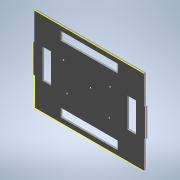
# Autodesk Inventor part: Level3
Saved by Autodesk Inventor 2020 (Build 240168000, 168)
## iProperties
Part Number: Level3
Material: Generic
Document SubType Name: Modeling
Designer: SBBA
Appearance: Default
Mass: 74.2606 g
Surface Area: 539.274 cm^2
Volume: 74.2606 cm^3
Density: 1 g/cm^3
Author: SBBA
Autodesk Inventor part; units mm, degrees
ref_plane "YZ Plane" through (0, 0, 0) normal (1, 0, 0) x (0, 1, 0)
ref_plane "XZ Plane" through (0, 0, 0) normal (0, 1, 0) x (-1, 0, 0)
ref_plane "XY Plane" through (0, 0, 0) normal (0, 0, 1) x (1, 0, 0)
sketch "Sketch1" plane through (0, 0, 0) normal (0, 0, 1) x (1, 0, 0)
  line L0 (-102.5157, 69.2842) -> (97.4843, 69.2842)
  line L1 (97.4843, 69.2842) -> (97.4843, -80.7158)
  line L2 (97.4843, -80.7158) -> (-102.5157, -80.7158)
  line L3 (-102.5157, -80.7158) -> (-102.5157, 69.2842)
  point P0 (0, 0)
  constraints: 8 end point, 2 parallel, 1 horizontal, 1 perpendicular
extrude "Extrusion1" add sketch "Sketch1" along normal blind 3
sketch "Sketch3" plane through (0, 0, 3) normal (0, 0, 1) x (1, 0, 0)
  point P0 (0, 0)
sketch "Sketch4" plane through (0, 0, 3) normal (0, 0, 1) x (1, 0, 0)
  line L0 (97.4843, 69.2842) -> (-102.5157, 69.2842) projected
  line L1 (-102.5157, 69.2842) -> (-99.5157, 69.2842)
  line L2 (-99.5157, 69.2842) -> (-99.5157, 19.2842)
  line L3 (-99.5157, 19.2842) -> (-102.5157, 19.2842)
  line L4 (-102.5157, 19.2842) -> (-102.5157, 69.2842)
  point P0 (0, 0)
  constraints: 8 end point, 2 parallel, 1 horizontal, 1 perpendicular
extrude "Extrusion2" cut sketch "Sketch4" against normal blind 3
sketch "Sketch5" plane through (0, 0, 3) normal (0, 0, 1) x (1, 0, 0)
  line L0 (97.4843, -80.7158) -> (94.4843, -80.7158)
  line L1 (94.4843, -80.7158) -> (94.4843, -30.7158)
  line L2 (94.4843, -30.7158) -> (97.4843, -30.7158)
  line L3 (97.4843, -30.7158) -> (97.4843, -80.7158)
  point P0 (0, 0)
  point P1 (-102.5157, -80.7158)
  dimension "d17" = 3
  dimension "d18" = 50
  constraints: 8 end point, 2 parallel, 1 horizontal, 1 perpendicular
  measures "d17" distance of L1.end L2.end
  measures "d18" distance of L2.end L0.start
extrude "Extrusion3" cut sketch "Sketch5" against normal blind 3
sketch "Sketch6" plane through (0, 0, 3) normal (0, 0, 1) x (1, 0, 0)
  line L0 (97.4843, -30.7158) -> (97.4843, 69.2842) projected
  line L1 (97.4843, 69.2842) -> (94.4843, 69.2842)
  line L2 (94.4843, 69.2842) -> (94.4843, 19.2842)
  line L3 (94.4843, 19.2842) -> (97.4843, 19.2842)
  line L4 (97.4843, 19.2842) -> (97.4843, 69.2842)
  point P0 (0, 0)
  dimension "d21" = 50
  dimension "d22" = 3
  constraints: 8 end point, 2 parallel, 1 horizontal, 1 perpendicular
  measures "d21" distance of L1.end L2.end
  measures "d22" distance of L0.end L1.end
extrude "Extrusion4" cut sketch "Sketch6" against normal blind 3
sketch "Sketch7" plane through (0, 0, 3) normal (0, 0, 1) x (1, 0, 0)
  line L0 (-102.5157, 19.2842) -> (-102.5157, -80.7158) projected
  line L1 (-102.5157, -80.7158) -> (-99.5157, -80.7158)
  line L2 (-99.5157, -80.7158) -> (-99.5157, -30.7158)
  line L3 (-99.5157, -30.7158) -> (-102.5157, -30.7158)
  line L4 (-102.5157, -30.7158) -> (-102.5157, -80.7158)
  point P0 (0, 0)
  dimension "d25" = 50
  dimension "d26" = 3
  constraints: 8 end point, 2 parallel, 1 horizontal, 1 perpendicular
  measures "d25" distance of L1.end L2.end
  measures "d26" distance of L2.end L3.end
extrude "Extrusion5" cut sketch "Sketch7" against normal blind 3
sketch "Sketch8" plane through (0, 0, 3) normal (0, 0, 1) x (1, 0, 0)
  line L0 (-102.5157, -30.7158) -> (-102.5157, 19.2842) projected
  line L1 (97.4843, -30.7158) -> (94.4843, -30.7158) projected
  line L2 (94.4843, -80.7158) -> (-99.5157, -80.7158) projected
  line L3 (-10.0157, -50.7158) -> (4.9843, -50.7158)
  line L4 (4.9843, -50.7158) -> (4.9843, -80.7158)
  line L5 (4.9843, -80.7158) -> (-10.0157, -80.7158)
  line L6 (-10.0157, -80.7158) -> (-10.0157, -50.7158)
  point P0 (0, 0)
  dimension "d32" = 15
  dimension "d33" = 30
  constraints: 8 end point, 2 parallel, 1 horizontal, 1 perpendicular, 1 point on line
  measures "d32" distance of L3.start L3.end
  measures "d33" distance of L3.end L4.end
extrude "Extrusion6" cut sketch "Sketch8" against normal blind 3
sketch "Sketch9" plane through (-10.0157, -80.7158, 3) normal (1, 0, 0) x (0, 0, -1)
  point P0 (3, 80.7158)
sketch "Sketch10" plane through (-10.0157, -50.7158, 3) normal (0, -1, 0) x (1, 0, 0)
  line L0 (15, 0) -> (15, -3) projected
  line L1 (15, -3) -> (0, -3) projected
  line L2 (15, 0) -> (0, 0)
  line L3 (0, 0) -> (0, -3)
  line L4 (0, -3) -> (15, -3)
  line L5 (15, -3) -> (15, 0)
  point P0 (10.0157, -3)
  constraints: 8 end point, 2 parallel, 1 horizontal, 1 perpendicular
extrude "Extrusion7" add sketch "Sketch10" along normal blind 30
sketch "Sketch11" plane through (0, 0, 3) normal (0, 0, 1) x (1, 0, 0)
  line L0 (94.4843, -80.7158) -> (-99.5157, -80.7158) projected
  line L1 (-99.5157, -80.7158) -> (-99.5157, -30.7158) projected
  line L2 (97.4843, 19.2842) -> (97.4843, -30.7158) projected
  line L3 (-102.5157, -30.7158) -> (-102.5157, 19.2842) projected
  line L4 (-99.5157, 69.2842) -> (94.4843, 69.2842) projected
  point P0 (0, 0)
sketch "Sketch12" plane through (0, 0, 3) normal (0, 0, 1) x (1, 0, 0)
  circle A0 centre (34.4088, 18.4314) radius 1.5
  circle A1 centre (33.1388, -29.8286) radius 1.5
  circle A2 centre (-41.7912, -29.8286) radius 1.5
  circle A3 centre (-48.1412, 18.4314) radius 1.5
  point P0 (0, 0)
  constraints: 4 centre point
extrude "Extrusion8" cut sketch "Sketch12" against normal blind 3
sketch "Sketch13" plane through (0, 0, 3) normal (0, 0, 1) x (1, 0, 0)
  line L0 (-99.5157, 69.2842) -> (94.4843, 69.2842) projected
  line L1 (-102.5157, -30.7158) -> (-102.5157, 19.2842) projected
  line L2 (94.4843, -80.7158) -> (-99.5157, -80.7158) projected
  line L3 (-85.4157, 20.4542) -> (-70.4157, 20.4542)
  line L4 (-70.4157, 20.4542) -> (-70.4157, -31.8858)
  line L5 (-70.4157, -31.8858) -> (-85.4157, -31.8858)
  line L6 (-85.4157, -31.8858) -> (-85.4157, 20.4542)
  line L7 (-53.3157, 45.7842) -> (48.2843, 45.7842)
  line L8 (48.2843, 45.7842) -> (48.2843, 60.7842)
  line L9 (48.2843, 60.7842) -> (-53.3157, 60.7842)
  line L10 (-53.3157, 60.7842) -> (-53.3157, 45.7842)
  line L11 (65.3843, 20.4542) -> (80.3843, 20.4542)
  line L12 (80.3843, 20.4542) -> (80.3843, -31.8858)
  line L13 (80.3843, -31.8858) -> (65.3843, -31.8858)
  line L14 (65.3843, -31.8858) -> (65.3843, 20.4542)
  line L15 (97.4843, -30.7158) -> (97.4843, 19.2842) projected
  line L16 (94.4843, 69.2842) -> (94.4843, 19.2842) projected
  line L17 (-99.5157, 19.2842) -> (-99.5157, 69.2842) projected
  line L18 (-53.3157, -72.2158) -> (48.2843, -72.2158)
  line L19 (48.2843, -72.2158) -> (48.2843, -57.2158)
  line L20 (48.2843, -57.2158) -> (-53.3157, -57.2158)
  line L21 (-53.3157, -57.2158) -> (-53.3157, -72.2158)
  line L22 (-99.5157, -30.7158) -> (-99.5157, -80.7158) projected
  line L23 (94.4843, -30.7158) -> (94.4843, -80.7158) projected
  point P0 (0, 0)
  constraints: 32 end point, 8 parallel, 4 horizontal, 4 perpendicular
extrude "Extrusion9" cut sketch "Sketch13" against normal blind 3
sketch "Sketch14" plane through (0, 0, 3) normal (0, 0, 1) x (1, 0, 0)
  point P0 (0, 0)
body "Solid1"
